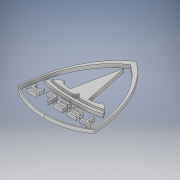
# Autodesk Inventor part: tesla
Saved by Autodesk Inventor 2019 (Build 230136000, 136)
## iProperties
Created: 2019-12-04
Part Number: tesla
Material: Generic
Document SubType Name: Modeling
Designer: Filip
Density: 1 g/cm^3
Appearance: Default
Author: Filip
Autodesk Inventor part; units mm, degrees
ref_plane "YZ Plane" through (0, 0, 0) normal (1, 0, 0) x (0, 1, 0)
ref_plane "XZ Plane" through (0, 0, 0) normal (0, 1, 0) x (-1, 0, 0)
ref_plane "XY Plane" through (0, 0, 0) normal (0, 0, 1) x (1, 0, 0)
sketch "Sketch1" plane through (0, 0, 0) normal (0, 1, 0) x (-1, 0, 0)
  arc A0 (11.1622, 39.9259) -> (12.132, 38.9612) centre (12.4853, 40.2861) ccw
  arc A1 (15.6628, 40.879) -> (16.6146, 41.8423) centre (15.2904, 42.1988) ccw
  arc A2 (15.7072, 42.756) -> (16.6146, 43.706) centre (15.2904, 44.0625) ccw
  arc A3 (11.1622, 41.8423) -> (12.1266, 40.879) centre (12.4853, 42.2025) ccw
  arc A4 (11.1622, 43.706) -> (12.0805, 42.756) centre (12.4853, 44.0662) ccw
  line L0 (12.1266, 40.879) -> (15.6628, 40.879)
  line L1 (12.0805, 42.756) -> (15.7072, 42.756)
  line L2 (11.1622, 39.9259) -> (16.6146, 39.9259)
  line L3 (11.1622, 41.8423) -> (16.6146, 41.8423)
  line L4 (11.1622, 43.706) -> (16.6146, 43.706)
  arc A5 (8.2724, 42.756) -> (9.1907, 43.706) centre (7.8676, 44.0662) ccw
  line L5 (6.6782, 38.9612) -> (6.6782, 42.756)
  line L6 (6.6782, 42.756) -> (8.2724, 42.756)
  line L7 (5.7339, 38.9612) -> (6.6782, 38.9612)
  line L8 (12.132, 38.9612) -> (15.6576, 38.9612)
  spline S0 degree 3 poles (21.4586, 50.9619) (20.7561, 50.9551) (18.8162, 50.9364) (15.6463, 50.6338) (12.4585, 49.9963) (9.7861, 49.2205) (7.7101, 48.5168) (5.5564, 47.5753) (3.4665, 46.5737) (1.7701, 45.5405) (0.9252, 44.9147) (0.6788, 44.7255) knots 0 0 0 0 3.193036 8.81673 14.444134 17.941513 21.46156 24.397967 28.620162 31.989333 33.401627 33.401627 33.401627 33.401627
  line L9 (21.4586, 50.9619) -> (20.7561, 50.9551) construction
  line L10 (20.7561, 50.9551) -> (18.8162, 50.9364) construction
  line L11 (18.8162, 50.9364) -> (15.6463, 50.6338) construction
  line L12 (15.6463, 50.6338) -> (12.4585, 49.9963) construction
  line L13 (12.4585, 49.9963) -> (9.7861, 49.2205) construction
  line L14 (9.7861, 49.2205) -> (7.7101, 48.5168) construction
  line L15 (7.7101, 48.5168) -> (5.5564, 47.5753) construction
  line L16 (5.5564, 47.5753) -> (3.4665, 46.5737) construction
  line L17 (3.4665, 46.5737) -> (1.7701, 45.5405) construction
  line L18 (1.7701, 45.5405) -> (0.9252, 44.9147) construction
  line L19 (0.9252, 44.9147) -> (0.6788, 44.7255) construction
  spline S1 degree 3 poles (21.4586, 51.5398) (20.7561, 51.5331) (18.8162, 51.5144) (15.6463, 51.2117) (12.4585, 50.5743) (9.7861, 49.7985) (7.7101, 49.0948) (5.5564, 48.1532) (3.4665, 47.1516) (1.5069, 45.9581) (0.4362, 45.1204) (-0.0451, 44.7319) knots 0 0 0 0 3.193036 8.81673 14.444134 17.941513 21.46156 24.397967 28.620162 31.989333 34.798673 34.798673 34.798673 34.798673
  line L20 (21.4586, 51.5398) -> (20.7561, 51.5331) construction
  line L21 (20.7561, 51.5331) -> (18.8162, 51.5144) construction
  line L22 (18.8162, 51.5144) -> (15.6463, 51.2117) construction
  line L23 (15.6463, 51.2117) -> (12.4585, 50.5743) construction
  line L24 (12.4585, 50.5743) -> (9.7861, 49.7985) construction
  line L25 (9.7861, 49.7985) -> (7.7101, 49.0948) construction
  line L26 (7.7101, 49.0948) -> (5.5564, 48.1532) construction
  line L27 (5.5564, 48.1532) -> (3.4665, 47.1516) construction
  line L28 (3.4665, 47.1516) -> (1.5069, 45.9581) construction
  line L29 (1.5069, 45.9581) -> (0.4362, 45.1204) construction
  line L30 (0.4362, 45.1204) -> (-0.0451, 44.7319) construction
  arc A6 (15.6576, 38.9612) -> (16.6146, 39.9259) centre (15.2904, 40.2824) ccw
  line L31 (23.257, 38.9618) -> (23.257, 38.9612)
  line L32 (24.1649, 41.8423) -> (24.1649, 38.9612)
  line L33 (23.257, 40.879) -> (23.257, 39.9259)
  line L34 (19.9315, 39.9259) -> (23.257, 39.9259)
  line L35 (19.9315, 42.756) -> (19.9315, 41.8423)
  line L36 (19.9315, 41.8423) -> (24.1649, 41.8423)
  line L37 (19.0032, 43.706) -> (19.0032, 40.879)
  line L38 (19.0032, 43.706) -> (24.1649, 43.706)
  line L39 (19.0032, 40.879) -> (23.257, 40.879)
  line L40 (18.7354, 38.9612) -> (24.1649, 38.9612)
  arc A7 (19.9315, 39.9259) -> (18.7354, 38.9612) centre (20.4205, 38.0959) ccw
  line L41 (19.9315, 42.756) -> (23.2471, 42.756)
  spline S2 degree 3 poles (36.9713, 33.2506) (37.2903, 33.704) (37.6122, 34.1554) (37.9345, 34.6065) knots 2.045296 2.045296 2.045296 2.045296 4.56531 4.56531 4.56531 4.56531
  line L42 (36.9713, 33.2506) -> (37.2903, 33.704) construction
  line L43 (37.2903, 33.704) -> (37.6122, 34.1554) construction
  line L44 (37.6122, 34.1554) -> (37.9345, 34.6065) construction
  spline S3 degree 3 poles (21.4586, 36.5616) (23.1459, 36.5381) (26.183, 36.4958) (30.2008, 36.1943) (33.5307, 35.7129) (35.9953, 35.1942) (37.4567, 34.7558) (37.9345, 34.6065) knots 0 0 0 0 7.669466 13.804429 18.296547 22.957419 25.232421 25.232421 25.232421 25.232421
  line L45 (21.4586, 36.5616) -> (23.1459, 36.5381) construction
  line L46 (23.1459, 36.5381) -> (26.183, 36.4958) construction
  line L47 (26.183, 36.4958) -> (30.2008, 36.1943) construction
  line L48 (30.2008, 36.1943) -> (33.5307, 35.7129) construction
  line L49 (33.5307, 35.7129) -> (35.9953, 35.1942) construction
  line L50 (35.9953, 35.1942) -> (37.4567, 34.7558) construction
  line L51 (37.4567, 34.7558) -> (37.9345, 34.6065) construction
  spline S4 degree 3 poles (21.4586, 35.1538) (22.8987, 35.1552) (25.3232, 35.1573) (28.6511, 34.9082) (31.6152, 34.4744) (34.374, 33.9514) (36.2053, 33.4625) (36.9713, 33.2506) knots 0 0 0 0 6.544078 11.01704 15.153003 20.156855 23.768247 23.768247 23.768247 23.768247
  line L52 (21.4586, 35.1538) -> (22.8987, 35.1552) construction
  line L53 (22.8987, 35.1552) -> (25.3232, 35.1573) construction
  line L54 (25.3232, 35.1573) -> (28.6511, 34.9082) construction
  line L55 (28.6511, 34.9082) -> (31.6152, 34.4744) construction
  line L56 (31.6152, 34.4744) -> (34.374, 33.9514) construction
  line L57 (34.374, 33.9514) -> (36.2053, 33.4625) construction
  line L58 (36.2053, 33.4625) -> (36.9713, 33.2506) construction
  spline S5 degree 3 poles (36.1984, 32.1439) (36.1122, 32.024) (35.8078, 31.62) (35.1245, 31.0306) (34.1638, 30.3906) (33.1209, 29.8807) (32.4045, 29.5987) (32.0649, 29.4716) knots 0.364731 0.364731 0.364731 0.364731 1.034928 2.664172 4.425816 6.277684 7.92563 7.92563 7.92563 7.92563
  line L59 (36.1984, 32.1439) -> (36.1122, 32.024) construction
  line L60 (36.1122, 32.024) -> (35.8078, 31.62) construction
  line L61 (35.8078, 31.62) -> (35.1245, 31.0306) construction
  line L62 (35.1245, 31.0306) -> (34.1638, 30.3906) construction
  line L63 (34.1638, 30.3906) -> (33.1209, 29.8807) construction
  line L64 (33.1209, 29.8807) -> (32.4045, 29.5987) construction
  line L65 (32.4045, 29.5987) -> (32.0649, 29.4716) construction
  line L66 (23.2328, 33.6071) -> (21.4586, 31.5742)
  spline S6 degree 3 poles (23.2328, 33.6071) (24.1252, 33.6197) (26.068, 33.6472) (29.4658, 33.4399) (32.9331, 33.0568) (35.2714, 32.4083) (36.1984, 32.1439) knots 0 0 0 0 4.05505 8.828209 15.472704 19.848815 19.848815 19.848815 19.848815
  line L67 (23.2328, 33.6071) -> (24.1252, 33.6197) construction
  line L68 (24.1252, 33.6197) -> (26.068, 33.6472) construction
  line L69 (26.068, 33.6472) -> (29.4658, 33.4399) construction
  line L70 (29.4658, 33.4399) -> (32.9331, 33.0568) construction
  line L71 (32.9331, 33.0568) -> (35.2714, 32.4083) construction
  line L72 (35.2714, 32.4083) -> (36.1984, 32.1439) construction
  line L73 (21.4586, 6.6382) -> (26.5701, 31.7392)
  spline S7 degree 3 poles (26.5701, 31.7392) (27.284, 31.729) (28.4836, 31.7107) (29.943, 31.4582) (30.866, 31.0777) (31.4703, 30.7194) (31.8929, 30.2653) (32.0023, 29.838) (32.0421, 29.6026) (32.0649, 29.4716) knots 0.039893 0.039893 0.039893 0.039893 3.283927 5.491546 6.716028 7.801422 8.675298 9.443739 9.761747 9.761747 9.761747 9.761747
  line L74 (26.5701, 31.7392) -> (27.284, 31.729) construction
  line L75 (27.284, 31.729) -> (28.4836, 31.7107) construction
  line L76 (28.4836, 31.7107) -> (29.943, 31.4582) construction
  line L77 (29.943, 31.4582) -> (30.866, 31.0777) construction
  line L78 (30.866, 31.0777) -> (31.4703, 30.7194) construction
  line L79 (31.4703, 30.7194) -> (31.8929, 30.2653) construction
  line L80 (31.8929, 30.2653) -> (32.0023, 29.838) construction
  line L81 (32.0023, 29.838) -> (32.0421, 29.6026) construction
  line L82 (32.0421, 29.6026) -> (32.0649, 29.4716) construction
  spline S8 degree 3 poles (21.4586, -0.0615) (21.698, 0.0967) (22.6847, 0.7569) (24.5171, 2.2096) (27.3457, 4.767) (30.2357, 8.0133) (33.4246, 12.4895) (36.7968, 18.5992) (39.9145, 26.8466) (41.8234, 34.7453) (42.6526, 40.7522) (42.8753, 43.5499) (42.9623, 44.7319) knots 0.560038 0.560038 0.560038 0.560038 1.86425 5.956382 11.172047 19.186039 25.65086 36.124233 50.807585 65.591245 72.961519 78.348003 78.348003 78.348003 78.348003
  line L83 (21.4586, -0.0615) -> (21.698, 0.0967) construction
  line L84 (21.698, 0.0967) -> (22.6847, 0.7569) construction
  line L85 (22.6847, 0.7569) -> (24.5171, 2.2096) construction
  line L86 (24.5171, 2.2096) -> (27.3457, 4.767) construction
  line L87 (27.3457, 4.767) -> (30.2357, 8.0133) construction
  line L88 (30.2357, 8.0133) -> (33.4246, 12.4895) construction
  line L89 (33.4246, 12.4895) -> (36.7968, 18.5992) construction
  line L90 (36.7968, 18.5992) -> (39.9145, 26.8466) construction
  line L91 (39.9145, 26.8466) -> (41.8234, 34.7453) construction
  line L92 (41.8234, 34.7453) -> (42.6526, 40.7522) construction
  line L93 (42.6526, 40.7522) -> (42.8753, 43.5499) construction
  line L94 (42.8753, 43.5499) -> (42.9623, 44.7319) construction
  line L95 (19.6844, 33.6071) -> (21.4586, 31.5742)
  line L96 (5.7339, 38.9612) -> (5.7339, 42.756)
  spline S9 degree 3 poles (16.3471, 31.7392) (15.6332, 31.729) (14.4336, 31.7107) (12.9742, 31.4582) (12.0512, 31.0777) (11.4469, 30.7194) (11.0243, 30.2653) (10.9149, 29.838) (10.8751, 29.6026) (10.8523, 29.4716) knots 0.039893 0.039893 0.039893 0.039893 3.283927 5.491546 6.716028 7.801422 8.675298 9.443739 9.761747 9.761747 9.761747 9.761747
  line L97 (16.3471, 31.7392) -> (15.6332, 31.729) construction
  line L98 (15.6332, 31.729) -> (14.4336, 31.7107) construction
  line L99 (14.4336, 31.7107) -> (12.9742, 31.4582) construction
  line L100 (12.9742, 31.4582) -> (12.0512, 31.0777) construction
  line L101 (12.0512, 31.0777) -> (11.4469, 30.7194) construction
  line L102 (11.4469, 30.7194) -> (11.0243, 30.2653) construction
  line L103 (11.0243, 30.2653) -> (10.9149, 29.838) construction
  line L104 (10.9149, 29.838) -> (10.8751, 29.6026) construction
  line L105 (10.8751, 29.6026) -> (10.8523, 29.4716) construction
  line L106 (4.157, 42.756) -> (5.7339, 42.756)
  spline S10 degree 3 poles (5.9459, 33.2506) (5.6269, 33.704) (5.3051, 34.1554) (4.9827, 34.6065) knots 2.045296 2.045296 2.045296 2.045296 4.56531 4.56531 4.56531 4.56531
  line L107 (5.9459, 33.2506) -> (5.6269, 33.704) construction
  line L108 (5.6269, 33.704) -> (5.3051, 34.1554) construction
  line L109 (5.3051, 34.1554) -> (4.9827, 34.6065) construction
  line L110 (3.2387, 43.706) -> (9.1907, 43.706)
  arc A8 (3.2387, 43.706) -> (4.157, 42.756) centre (4.5618, 44.0662) ccw
  spline S11 degree 3 poles (6.7188, 32.1439) (6.805, 32.024) (7.1094, 31.62) (7.7927, 31.0306) (8.7534, 30.3906) (9.7963, 29.8807) (10.5127, 29.5987) (10.8523, 29.4716) knots 0.364731 0.364731 0.364731 0.364731 1.034928 2.664172 4.425816 6.277684 7.92563 7.92563 7.92563 7.92563
  line L111 (6.7188, 32.1439) -> (6.805, 32.024) construction
  line L112 (6.805, 32.024) -> (7.1094, 31.62) construction
  line L113 (7.1094, 31.62) -> (7.7927, 31.0306) construction
  line L114 (7.7927, 31.0306) -> (8.7534, 30.3906) construction
  line L115 (8.7534, 30.3906) -> (9.7963, 29.8807) construction
  line L116 (9.7963, 29.8807) -> (10.5127, 29.5987) construction
  line L117 (10.5127, 29.5987) -> (10.8523, 29.4716) construction
  spline S12 degree 3 poles (19.6844, 33.6071) (18.792, 33.6197) (16.8492, 33.6472) (13.4514, 33.4399) (9.9841, 33.0568) (7.6458, 32.4083) (6.7188, 32.1439) knots 0 0 0 0 4.05505 8.828209 15.472704 19.848815 19.848815 19.848815 19.848815
  line L118 (19.6844, 33.6071) -> (18.792, 33.6197) construction
  line L119 (18.792, 33.6197) -> (16.8492, 33.6472) construction
  line L120 (16.8492, 33.6472) -> (13.4514, 33.4399) construction
  line L121 (13.4514, 33.4399) -> (9.9841, 33.0568) construction
  line L122 (9.9841, 33.0568) -> (7.6458, 32.4083) construction
  line L123 (7.6458, 32.4083) -> (6.7188, 32.1439) construction
  spline S13 degree 3 poles (21.4586, 35.1538) (20.0185, 35.1552) (17.594, 35.1573) (14.2661, 34.9082) (11.302, 34.4744) (8.5432, 33.9514) (6.7119, 33.4625) (5.9459, 33.2506) knots 0 0 0 0 6.544078 11.01704 15.153003 20.156855 23.768247 23.768247 23.768247 23.768247
  line L124 (21.4586, 35.1538) -> (20.0185, 35.1552) construction
  line L125 (20.0185, 35.1552) -> (17.594, 35.1573) construction
  line L126 (17.594, 35.1573) -> (14.2661, 34.9082) construction
  line L127 (14.2661, 34.9082) -> (11.302, 34.4744) construction
  line L128 (11.302, 34.4744) -> (8.5432, 33.9514) construction
  line L129 (8.5432, 33.9514) -> (6.7119, 33.4625) construction
  line L130 (6.7119, 33.4625) -> (5.9459, 33.2506) construction
  spline S14 degree 3 poles (21.4586, 36.5616) (19.7713, 36.5381) (16.7342, 36.4958) (12.7164, 36.1943) (9.3865, 35.7129) (6.9219, 35.1942) (5.4605, 34.7558) (4.9827, 34.6065) knots 0 0 0 0 7.669466 13.804429 18.296547 22.957419 25.232421 25.232421 25.232421 25.232421
  line L131 (21.4586, 36.5616) -> (19.7713, 36.5381) construction
  line L132 (19.7713, 36.5381) -> (16.7342, 36.4958) construction
  line L133 (16.7342, 36.4958) -> (12.7164, 36.1943) construction
  line L134 (12.7164, 36.1943) -> (9.3865, 35.7129) construction
  line L135 (9.3865, 35.7129) -> (6.9219, 35.1942) construction
  line L136 (6.9219, 35.1942) -> (5.4605, 34.7558) construction
  line L137 (5.4605, 34.7558) -> (4.9827, 34.6065) construction
  spline S15 degree 3 poles (21.4586, 3.0192) (21.7096, 3.1952) (22.4574, 3.722) (23.633, 4.5923) (25.2375, 5.9285) (27.1129, 7.6277) (30.1948, 10.8387) (33.7857, 15.9291) (37.3139, 22.9396) (39.7414, 30.0279) (41.287, 36.7041) (42.0796, 41.4373) (42.2142, 44.1109) (42.2384, 44.7255) knots 0.528542 0.528542 0.528542 0.528542 1.921958 4.68642 7.174129 11.410102 16.184154 27.379679 39.559638 51.755042 61.330303 70.704771 73.499884 73.499884 73.499884 73.499884
  line L138 (21.4586, 3.0192) -> (21.7096, 3.1952) construction
  line L139 (21.7096, 3.1952) -> (22.4574, 3.722) construction
  line L140 (22.4574, 3.722) -> (23.633, 4.5923) construction
  line L141 (23.633, 4.5923) -> (25.2375, 5.9285) construction
  line L142 (25.2375, 5.9285) -> (27.1129, 7.6277) construction
  line L143 (27.1129, 7.6277) -> (30.1948, 10.8387) construction
  line L144 (30.1948, 10.8387) -> (33.7857, 15.9291) construction
  line L145 (33.7857, 15.9291) -> (37.3139, 22.9396) construction
  line L146 (37.3139, 22.9396) -> (39.7414, 30.0279) construction
  line L147 (39.7414, 30.0279) -> (41.287, 36.7041) construction
  line L148 (41.287, 36.7041) -> (42.0796, 41.4373) construction
  line L149 (42.0796, 41.4373) -> (42.2142, 44.1109) construction
  line L150 (42.2142, 44.1109) -> (42.2384, 44.7255) construction
  line L151 (21.4586, 6.6382) -> (16.3471, 31.7392)
  spline S16 degree 3 poles (21.4586, 3.0192) (21.2076, 3.1952) (20.4598, 3.722) (19.2842, 4.5923) (17.6797, 5.9285) (15.8043, 7.6277) (12.7224, 10.8387) (9.1315, 15.9291) (5.6033, 22.9396) (3.1758, 30.0279) (1.6303, 36.7041) (0.8376, 41.4373) (0.703, 44.1109) (0.6788, 44.7255) knots 0.528542 0.528542 0.528542 0.528542 1.921958 4.68642 7.174129 11.410102 16.184154 27.379679 39.559638 51.755042 61.330303 70.704771 73.499884 73.499884 73.499884 73.499884
  line L152 (21.4586, 3.0192) -> (21.2076, 3.1952) construction
  line L153 (21.2076, 3.1952) -> (20.4598, 3.722) construction
  line L154 (20.4598, 3.722) -> (19.2842, 4.5923) construction
  line L155 (19.2842, 4.5923) -> (17.6797, 5.9285) construction
  line L156 (17.6797, 5.9285) -> (15.8043, 7.6277) construction
  line L157 (15.8043, 7.6277) -> (12.7224, 10.8387) construction
  line L158 (12.7224, 10.8387) -> (9.1315, 15.9291) construction
  line L159 (9.1315, 15.9291) -> (5.6033, 22.9396) construction
  line L160 (5.6033, 22.9396) -> (3.1758, 30.0279) construction
  line L161 (3.1758, 30.0279) -> (1.6303, 36.7041) construction
  line L162 (1.6303, 36.7041) -> (0.8376, 41.4373) construction
  line L163 (0.8376, 41.4373) -> (0.703, 44.1109) construction
  line L164 (0.703, 44.1109) -> (0.6788, 44.7255) construction
  spline S17 degree 3 poles (21.4586, -0.0615) (21.2192, 0.0967) (20.2325, 0.7569) (18.4001, 2.2096) (15.5715, 4.767) (12.6815, 8.0133) (9.4926, 12.4895) (6.1204, 18.5992) (3.0027, 26.8466) (1.0938, 34.7453) (0.2646, 40.7522) (0.0419, 43.5499) (-0.0451, 44.7319) knots 0.560038 0.560038 0.560038 0.560038 1.86425 5.956382 11.172047 19.186039 25.65086 36.124233 50.807585 65.591245 72.961519 78.348003 78.348003 78.348003 78.348003
  line L165 (21.4586, -0.0615) -> (21.2192, 0.0967) construction
  line L166 (21.2192, 0.0967) -> (20.2325, 0.7569) construction
  line L167 (20.2325, 0.7569) -> (18.4001, 2.2096) construction
  line L168 (18.4001, 2.2096) -> (15.5715, 4.767) construction
  line L169 (15.5715, 4.767) -> (12.6815, 8.0133) construction
  line L170 (12.6815, 8.0133) -> (9.4926, 12.4895) construction
  line L171 (9.4926, 12.4895) -> (6.1204, 18.5992) construction
  line L172 (6.1204, 18.5992) -> (3.0027, 26.8466) construction
  line L173 (3.0027, 26.8466) -> (1.0938, 34.7453) construction
  line L174 (1.0938, 34.7453) -> (0.2646, 40.7522) construction
  line L175 (0.2646, 40.7522) -> (0.0419, 43.5499) construction
  line L176 (0.0419, 43.5499) -> (-0.0451, 44.7319) construction
  arc A9 (23.2471, 42.756) -> (24.1649, 43.706) centre (22.8417, 44.066) ccw
  line L177 (26.6035, 43.706) -> (26.6035, 38.9612)
  line L178 (27.5415, 43.706) -> (27.5415, 39.9259)
  line L179 (26.6035, 43.706) -> (27.5415, 43.706)
  line L180 (26.6035, 38.9612) -> (30.6881, 38.9612)
  line L181 (27.5415, 39.9259) -> (31.6573, 39.9259)
  arc A10 (30.6881, 38.9612) -> (31.6573, 39.9259) centre (30.3341, 40.286) ccw
  line L182 (33.7717, 41.8423) -> (33.7717, 38.9612)
  arc A11 (33.6371, 43.706) -> (34.5826, 42.756) centre (34.8737, 43.9913) ccw
  line L183 (34.7099, 40.879) -> (34.7099, 38.9612)
  line L184 (33.7717, 38.9612) -> (34.7099, 38.9612)
  line L185 (38.0243, 40.879) -> (38.0243, 38.9612)
  line L186 (38.9632, 41.8423) -> (38.9632, 38.9612)
  line L187 (38.0243, 38.9612) -> (38.9632, 38.9612)
  line L188 (34.7099, 40.879) -> (38.0243, 40.879)
  line L189 (34.5826, 42.756) -> (38.029, 42.756)
  line L190 (33.7717, 41.8423) -> (38.9632, 41.8423)
  arc A12 (38.029, 42.756) -> (39.0868, 43.706) centre (37.8554, 44.0133) ccw
  line L191 (33.6371, 43.706) -> (39.0868, 43.706)
  spline S18 degree 3 poles (21.4586, 51.5398) (22.1612, 51.5331) (24.101, 51.5144) (27.271, 51.2117) (30.4588, 50.5743) (33.1311, 49.7985) (35.2071, 49.0948) (37.3608, 48.1532) (39.4507, 47.1516) (41.4103, 45.9581) (42.481, 45.1204) (42.9623, 44.7319) knots 0 0 0 0 3.193036 8.81673 14.444134 17.941513 21.46156 24.397967 28.620162 31.989333 34.798673 34.798673 34.798673 34.798673
  line L192 (21.4586, 51.5398) -> (22.1612, 51.5331) construction
  line L193 (22.1612, 51.5331) -> (24.101, 51.5144) construction
  line L194 (24.101, 51.5144) -> (27.271, 51.2117) construction
  line L195 (27.271, 51.2117) -> (30.4588, 50.5743) construction
  line L196 (30.4588, 50.5743) -> (33.1311, 49.7985) construction
  line L197 (33.1311, 49.7985) -> (35.2071, 49.0948) construction
  line L198 (35.2071, 49.0948) -> (37.3608, 48.1532) construction
  line L199 (37.3608, 48.1532) -> (39.4507, 47.1516) construction
  line L200 (39.4507, 47.1516) -> (41.4103, 45.9581) construction
  line L201 (41.4103, 45.9581) -> (42.481, 45.1204) construction
  line L202 (42.481, 45.1204) -> (42.9623, 44.7319) construction
  spline S19 degree 3 poles (21.4586, 50.9619) (22.1612, 50.9551) (24.101, 50.9364) (27.271, 50.6338) (30.4588, 49.9963) (33.1311, 49.2205) (35.2071, 48.5168) (37.3608, 47.5753) (39.4507, 46.5737) (41.1471, 45.5405) (41.992, 44.9147) (42.2384, 44.7255) knots 0 0 0 0 3.193036 8.81673 14.444134 17.941513 21.46156 24.397967 28.620162 31.989333 33.401627 33.401627 33.401627 33.401627
  line L203 (21.4586, 50.9619) -> (22.1612, 50.9551) construction
  line L204 (22.1612, 50.9551) -> (24.101, 50.9364) construction
  line L205 (24.101, 50.9364) -> (27.271, 50.6338) construction
  line L206 (27.271, 50.6338) -> (30.4588, 49.9963) construction
  line L207 (30.4588, 49.9963) -> (33.1311, 49.2205) construction
  line L208 (33.1311, 49.2205) -> (35.2071, 48.5168) construction
  line L209 (35.2071, 48.5168) -> (37.3608, 47.5753) construction
  line L210 (37.3608, 47.5753) -> (39.4507, 46.5737) construction
  line L211 (39.4507, 46.5737) -> (41.1471, 45.5405) construction
  line L212 (41.1471, 45.5405) -> (41.992, 44.9147) construction
  line L213 (41.992, 44.9147) -> (42.2384, 44.7255) construction
  point P0 (0, 0)
  constraints: 84 end point, 26 point on circle, 13 centre point, 1 point on line, 60 other
extrude "Extrusion1" add sketch "Sketch1" along normal blind 2
body "Solid1"
